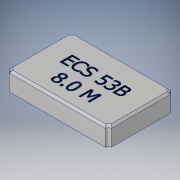
# Autodesk Inventor part: Crystal_ECX-42
Saved by Autodesk Inventor 2018 (Build 220112000, 112)
## iProperties
Created: 2016-08-15
Part Number: Crystal_ECX-42
Material: Aluminum 6061
Document SubType Name: Modeling
Designer: Bradley
Density: 2.7 g/cm^3
Appearance: Aluminum - Flat
Author: Bradley
Autodesk Inventor part; units mm, degrees
ref_plane "YZ Plane" through (0, 0, 0) normal (1, 0, 0) x (0, 1, 0)
ref_plane "XZ Plane" through (0, 0, 0) normal (0, 1, 0) x (-1, 0, 0)
ref_plane "XY Plane" through (0, 0, 0) normal (0, 0, 1) x (1, 0, 0)
sketch "Sketch1" plane through (0, 0, 0) normal (0, 1, 0) x (-1, 0, 0)
  line L0 (-2.5, 1.6) -> (2.5, 1.6)
  line L1 (2.5, 1.6) -> (2.5, -1.6)
  line L2 (2.5, -1.6) -> (-2.5, -1.6)
  line L3 (-2.5, -1.6) -> (-2.5, 1.6)
  line L4 (-2.5, 1.6) -> (2.5, -1.6) construction
  line L5 (2.5, 1.6) -> (-2.5, -1.6) construction
  arc A0 (2.5, -1.45) -> (2.35, -1.6) centre (2.5, -1.6) ccw
  arc A1 (-2.35, -1.6) -> (-2.5, -1.45) centre (-2.5, -1.6) ccw
  arc A2 (-2.5, 1.45) -> (-2.35, 1.6) centre (-2.5, 1.6) ccw
  arc A3 (2.35, 1.6) -> (2.5, 1.45) centre (2.5, 1.6) ccw
  point P0 (0, 0)
  dimension "d0" = 5
  dimension "d1" = 3.2
  dimension "d4" = 0.15
  constraints: 12 end point, 8 point on circle, 8 point on line, 4 centre point, 4 coincident, 3 equal radius, 2 midpoint, 2 parallel, 1 horizontal, 1 perpendicular
  measures "d0" distance of L1.end L2.end
  measures "d1" distance of L0.end L1.end
  measures "d4" radius of A0
extrude "Extrusion1" add sketch "Sketch1" along normal mid plane 0.9 contours L0 A3 L1 A0 L2 A1 L3 A2
chamfer "Chamfer1" distance 0.1 angle 45 8 edges at (0, 0.45, 1.6) (-2.3939, 0.45, 1.4939) (-2.5, 0.45, 0) (-2.3939, 0.45, -1.4939) (0, 0.45, -1.6) (2.3939, 0.45, -1.4939) (2.5, 0.45, 0) (2.3939, 0.45, 1.4939)
sketch "Sketch2" plane through (0, -0.45, 0) normal (0, -1, 0) x (1, 0, 0)
  line L0 (-2.5, 1.45) -> (-2.5, -1.45) projected
  arc A0 (-2.35, -1.6) -> (-2.5, -1.45) centre (-2.5, -1.6) ccw projected
  line L1 (-2.35, -1.6) -> (2.35, -1.6) projected
  arc A1 (2.5, -1.45) -> (2.35, -1.6) centre (2.5, -1.6) ccw projected
  line L2 (2.5, -1.45) -> (2.5, 1.45) projected
  arc A2 (2.35, 1.6) -> (2.5, 1.45) centre (2.5, 1.6) ccw projected
  line L3 (2.35, 1.6) -> (-2.35, 1.6) projected
  arc A3 (-2.5, 1.45) -> (-2.35, 1.6) centre (-2.5, 1.6) ccw projected
  arc A4 (-2.35, -1.6) -> (-2.5, -1.45) centre (-2.5, -1.6) ccw projected
  line L4 (-2.4612, -1.4551) -> (-2.4, -1.3939)
  line L5 (-2.4, 1.3939) -> (-2.4612, 1.4551)
  arc A5 (-2.5, 1.45) -> (-2.35, 1.6) centre (-2.5, 1.6) ccw projected
  line L6 (-2.3551, 1.5612) -> (-2.2939, 1.5)
  line L7 (-2.2939, 1.5) -> (-1.3, 1.5)
  line L8 (-1.3, -1.5) -> (-2.2939, -1.5)
  line L9 (-2.2939, -1.5) -> (-2.3551, -1.5612)
  arc A6 (2.35, 1.6) -> (2.5, 1.45) centre (2.5, 1.6) ccw projected
  line L10 (2.3551, 1.5612) -> (2.2939, 1.5)
  line L11 (2.2939, 1.5) -> (1.3, 1.5)
  line L12 (1.3, -1.5) -> (2.2939, -1.5)
  line L13 (2.2939, -1.5) -> (2.3551, -1.5612)
  arc A7 (2.5, -1.45) -> (2.35, -1.6) centre (2.5, -1.6) ccw projected
  line L14 (2.4612, -1.4551) -> (2.4, -1.3939)
  line L15 (2.4, 1.3939) -> (2.4612, 1.4551)
  line L16 (-2.5, 1.6) -> (-2.3939, 1.4939) construction
  line L17 (2.35, 1.6) -> (-2.35, 1.6) construction
  line L18 (-2.5, -1.6) -> (-2.3939, -1.4939) construction
  line L19 (-2.4, 1.3939) -> (-2.4, 0.7)
  line L20 (-2.4, 0.7) -> (-1.3, 0.7)
  line L21 (-1.3, 0.7) -> (-1.3, 1.5)
  line L22 (-2.4, -1.3939) -> (-2.4, -0.7)
  line L23 (-2.4, -0.7) -> (-1.3, -0.7)
  line L24 (-1.3, -0.7) -> (-1.3, -1.5)
  line L25 (2.4, -1.3939) -> (2.4, -0.7)
  line L26 (2.4, -0.7) -> (1.3, -0.7)
  line L27 (1.3, -0.7) -> (1.3, -1.5)
  line L28 (2.4, 1.3939) -> (2.4, 0.7)
  line L29 (2.4, 0.7) -> (1.3, 0.7)
  line L30 (1.3, 1.5) -> (1.3, 0.7)
  point P0 (0, 0)
  dimension "d9" = 0.15
  dimension "d17" = 0.8
  dimension "d20" = 1.1
  dimension "d22" = 0.1
  constraints: 52 end point, 15 equal length, 15 point on circle, 9 point on line, 8 parallel, 8 perpendicular, 1 collinear, 1 vertical, 1 other
  measures "d9" distance between parallel lines of L5 L6
  measures "d17" distance of L11.end L29.end
  measures "d20" distance of L28.end L29.end
  measures "d22" distance between parallel lines of L0 L19
sketch "Sketch3" plane through (0, 0.45, 0) normal (0, 1, 0) x (1, 0, 0)
  line L0 (-2.2709, 1.5) -> (2.2709, 1.5) projected
  arc A0 (-2.4, 1.3709) -> (-2.2709, 1.5) centre (-2.5, 1.6) ccw projected
  line L1 (-2.4, -1.3709) -> (-2.4, 1.3709) projected
  arc A1 (-2.2709, -1.5) -> (-2.4, -1.3709) centre (-2.5, -1.6) ccw projected
  line L2 (2.2709, -1.5) -> (-2.2709, -1.5) projected
  arc A2 (2.4, -1.3709) -> (2.2709, -1.5) centre (2.5, -1.6) ccw projected
  line L3 (2.4, 1.3709) -> (2.4, -1.3709) projected
  arc A3 (2.2709, 1.5) -> (2.4, 1.3709) centre (2.5, 1.6) ccw projected
  line L4 (2.4, 1.3709) -> (2.4, -1.3709) construction
  line L5 (2.4, 0) -> (-2.4, 0) construction
  line L6 (-1.4703, 0) -> (-1.4703, 0.6)
  line L7 (-1.4703, 0.6) -> (-1.095, 0.6)
  line L8 (-1.095, 0.6) -> (-1.095, 0.529)
  line L9 (-1.095, 0.529) -> (-1.3906, 0.529)
  line L10 (-1.3906, 0.529) -> (-1.3906, 0.3647)
  line L11 (-1.3906, 0.3647) -> (-1.1149, 0.3647)
  line L12 (-1.1149, 0.3647) -> (-1.1149, 0.2937)
  line L13 (-1.1149, 0.2937) -> (-1.3906, 0.2937)
  line L14 (-1.3906, 0.2937) -> (-1.3906, 0.071)
  line L15 (-1.3906, 0.071) -> (-1.095, 0.071)
  line L16 (-1.095, 0.071) -> (-1.095, 0)
  line L17 (-1.095, 0) -> (-1.4703, 0)
  spline S0 degree 2 poles (-0.7731, -0.0107) (-0.8314, -0.0107) (-0.9301, 0.0287) (-0.9661, 0.0681) knots 0 0 0 1 2 2 2
  spline S1 degree 2 poles (-0.9661, 0.0681) (-1.0021, 0.107) (-1.0415, 0.2237) (-1.0415, 0.2995) knots 0 0 0 1 2 2 2
  spline S2 degree 2 poles (-1.0415, 0.2995) (-1.0415, 0.3749) (-1.0031, 0.4867) (-0.9666, 0.528) knots 0 0 0 1 2 2 2
  spline S3 degree 2 poles (-0.9666, 0.528) (-0.9306, 0.5684) (-0.8324, 0.6107) (-0.7716, 0.6107) knots 0 0 0 1 2 2 2
  spline S4 degree 2 poles (-0.7716, 0.6107) (-0.7415, 0.6107) (-0.6885, 0.6019) (-0.6661, 0.5951) knots 0 0 0 1 2 2 2
  spline S5 degree 2 poles (-0.6661, 0.5951) (-0.6467, 0.5888) (-0.6063, 0.5708) (-0.5864, 0.5601) knots 0 0 0 1 2 2 2
  line L18 (-0.5864, 0.5601) -> (-0.5864, 0.4639)
  line L19 (-0.5864, 0.4639) -> (-0.5927, 0.4639)
  spline S6 degree 2 poles (-0.5927, 0.4639) (-0.6034, 0.4736) (-0.6365, 0.5008) (-0.6603, 0.5139) knots 0 0 0 1 2 2 2
  spline S7 degree 2 poles (-0.6603, 0.5139) (-0.6831, 0.5266) (-0.7371, 0.5426) (-0.7721, 0.5426) knots 0 0 0 1 2 2 2
  spline S8 degree 2 poles (-0.7721, 0.5426) (-0.8105, 0.5426) (-0.8791, 0.511) (-0.9049, 0.4809) knots 0 0 0 1 2 2 2
  spline S9 degree 2 poles (-0.9049, 0.4809) (-0.9301, 0.4502) (-0.9583, 0.3574) (-0.9583, 0.2995) knots 0 0 0 1 2 2 2
  spline S10 degree 2 poles (-0.9583, 0.2995) (-0.9583, 0.2378) (-0.9287, 0.1488) (-0.9029, 0.1182) knots 0 0 0 1 2 2 2
  spline S11 degree 2 poles (-0.9029, 0.1182) (-0.8776, 0.0885) (-0.81, 0.0583) (-0.7721, 0.0583) knots 0 0 0 1 2 2 2
  spline S12 degree 2 poles (-0.7721, 0.0583) (-0.7376, 0.0583) (-0.6788, 0.0754) (-0.6559, 0.088) knots 0 0 0 1 2 2 2
  spline S13 degree 2 poles (-0.6559, 0.088) (-0.634, 0.1006) (-0.6015, 0.1269) (-0.5922, 0.1361) knots 0 0 0 1 2 2 2
  line L20 (-0.5922, 0.1361) -> (-0.5864, 0.1361)
  line L21 (-0.5864, 0.1361) -> (-0.5864, 0.0408)
  spline S14 degree 2 poles (-0.5864, 0.0408) (-0.6063, 0.0316) (-0.6413, 0.0146) (-0.6661, 0.0068) knots 0 0 0 1 2 2 2
  spline S15 degree 2 poles (-0.6661, 0.0068) (-0.6924, -0.0019) (-0.7371, -0.0107) (-0.7731, -0.0107) knots 0 0 0 1 2 2 2
  spline S16 degree 2 poles (-0.3447, -0.0107) (-0.4099, -0.0107) (-0.5013, 0.0165) (-0.5417, 0.036) knots 0 0 0 1 2 2 2
  line L22 (-0.5417, 0.036) -> (-0.5417, 0.1361)
  line L23 (-0.5417, 0.1361) -> (-0.5358, 0.1361)
  spline S17 degree 2 poles (-0.5358, 0.1361) (-0.4964, 0.0992) (-0.3968, 0.0583) (-0.3506, 0.0583) knots 0 0 0 1 2 2 2
  spline S18 degree 2 poles (-0.3506, 0.0583) (-0.2844, 0.0583) (-0.2169, 0.1133) (-0.2169, 0.1585) knots 0 0 0 1 2 2 2
  spline S19 degree 2 poles (-0.2169, 0.1585) (-0.2169, 0.1945) (-0.2524, 0.2392) (-0.2908, 0.2504) knots 0 0 0 1 2 2 2
  spline S20 degree 2 poles (-0.2908, 0.2504) (-0.3185, 0.2582) (-0.3647, 0.2689) (-0.3992, 0.2776) knots 0 0 0 1 2 2 2
  spline S21 degree 2 poles (-0.3992, 0.2776) (-0.4303, 0.2859) (-0.4794, 0.3107) (-0.4984, 0.3306) knots 0 0 0 1 2 2 2
  spline S22 degree 2 poles (-0.4984, 0.3306) (-0.5169, 0.3506) (-0.5373, 0.4041) (-0.5373, 0.4391) knots 0 0 0 1 2 2 2
  spline S23 degree 2 poles (-0.5373, 0.4391) (-0.5373, 0.512) (-0.4235, 0.6107) (-0.3355, 0.6107) knots 0 0 0 1 2 2 2
  spline S24 degree 2 poles (-0.3355, 0.6107) (-0.2849, 0.6107) (-0.1955, 0.5908) (-0.1571, 0.5718) knots 0 0 0 1 2 2 2
  line L24 (-0.1571, 0.5718) -> (-0.1571, 0.4765)
  line L25 (-0.1571, 0.4765) -> (-0.1629, 0.4765)
  spline S25 degree 2 poles (-0.1629, 0.4765) (-0.1916, 0.5028) (-0.281, 0.5417) (-0.3301, 0.5417) knots 0 0 0 1 2 2 2
  spline S26 degree 2 poles (-0.3301, 0.5417) (-0.3856, 0.5417) (-0.4541, 0.4896) (-0.4541, 0.4473) knots 0 0 0 1 2 2 2
  spline S27 degree 2 poles (-0.4541, 0.4473) (-0.4541, 0.4094) (-0.4138, 0.3642) (-0.3759, 0.354) knots 0 0 0 1 2 2 2
  spline S28 degree 2 poles (-0.3759, 0.354) (-0.3506, 0.3472) (-0.2771, 0.3297) (-0.2528, 0.3224) knots 0 0 0 1 2 2 2
  spline S29 degree 2 poles (-0.2528, 0.3224) (-0.1911, 0.3034) (-0.1337, 0.2271) (-0.1337, 0.1712) knots 0 0 0 1 2 2 2
  spline S30 degree 2 poles (-0.1337, 0.1712) (-0.1337, 0.1357) (-0.1624, 0.0676) (-0.1882, 0.0438) knots 0 0 0 1 2 2 2
  spline S31 degree 2 poles (-0.1882, 0.0438) (-0.2169, 0.0175) (-0.2898, -0.0107) (-0.3447, -0.0107) knots 0 0 0 1 2 2 2
  spline S32 degree 2 poles (0.5519, 0.1906) (0.5519, 0.1473) (0.5241, 0.0734) (0.4989, 0.0462) knots 0 0 0 1 2 2 2
  spline S33 degree 2 poles (0.4989, 0.0462) (0.4736, 0.019) (0.3982, -0.0126) (0.3515, -0.0126) knots 0 0 0 1 2 2 2
  spline S34 degree 2 poles (0.3515, -0.0126) (0.3088, -0.0126) (0.2251, 0.0063) (0.1945, 0.0214) knots 0 0 0 1 2 2 2
  line L26 (0.1945, 0.0214) -> (0.1945, 0.1065)
  line L27 (0.1945, 0.1065) -> (0.2003, 0.1065)
  spline S35 degree 2 poles (0.2003, 0.1065) (0.2096, 0.0997) (0.2441, 0.0822) (0.265, 0.0744) knots 0 0 0 1 2 2 2
  spline S36 degree 2 poles (0.265, 0.0744) (0.2888, 0.0661) (0.3282, 0.0569) (0.353, 0.0569) knots 0 0 0 1 2 2 2
  spline S37 degree 2 poles (0.353, 0.0569) (0.3773, 0.0569) (0.423, 0.0744) (0.4395, 0.0934) knots 0 0 0 1 2 2 2
  spline S38 degree 2 poles (0.4395, 0.0934) (0.4546, 0.1113) (0.4702, 0.159) (0.4702, 0.1911) knots 0 0 0 1 2 2 2
  spline S39 degree 2 poles (0.4702, 0.1911) (0.4702, 0.2232) (0.4527, 0.264) (0.4361, 0.2776) knots 0 0 0 1 2 2 2
  spline S40 degree 2 poles (0.4361, 0.2776) (0.4191, 0.2927) (0.3686, 0.3053) (0.3379, 0.3053) knots 0 0 0 1 2 2 2
  spline S41 degree 2 poles (0.3379, 0.3053) (0.3049, 0.3053) (0.2392, 0.2951) (0.2193, 0.2908) knots 0 0 0 1 2 2 2
  line L28 (0.2193, 0.2908) -> (0.2193, 0.6)
  line L29 (0.2193, 0.6) -> (0.5485, 0.6)
  line L30 (0.5485, 0.6) -> (0.5485, 0.5295)
  line L31 (0.5485, 0.5295) -> (0.2966, 0.5295)
  line L32 (0.2966, 0.5295) -> (0.2966, 0.3695)
  spline S42 degree 2 poles (0.2966, 0.3695) (0.3112, 0.3715) (0.3394, 0.3729) (0.3511, 0.3729) knots 0 0 0 1 2 2 2
  spline S43 degree 2 poles (0.3511, 0.3729) (0.3972, 0.3729) (0.4609, 0.3579) (0.4901, 0.3355) knots 0 0 0 1 2 2 2
  spline S44 degree 2 poles (0.4901, 0.3355) (0.5198, 0.3131) (0.5519, 0.2451) (0.5519, 0.1906) knots 0 0 0 1 2 2 2
  spline S45 degree 2 poles (0.8003, 0.5431) (0.7784, 0.5431) (0.7352, 0.5324) (0.7143, 0.5241) knots 0 0 0 1 2 2 2
  spline S46 degree 2 poles (0.7143, 0.5241) (0.6948, 0.5159) (0.6661, 0.4984) (0.6549, 0.4906) knots 0 0 0 1 2 2 2
  line L33 (0.6549, 0.4906) -> (0.6501, 0.4906)
  line L34 (0.6501, 0.4906) -> (0.6501, 0.5757)
  spline S47 degree 2 poles (0.6501, 0.5757) (0.6763, 0.5898) (0.7663, 0.6126) (0.8066, 0.6126) knots 0 0 0 1 2 2 2
  spline S48 degree 2 poles (0.8066, 0.6126) (0.8475, 0.6126) (0.9083, 0.5961) (0.9331, 0.5786) knots 0 0 0 1 2 2 2
  spline S49 degree 2 poles (0.9331, 0.5786) (0.9593, 0.5596) (0.9865, 0.5047) (0.9865, 0.4677) knots 0 0 0 1 2 2 2
  spline S50 degree 2 poles (0.9865, 0.4677) (0.9865, 0.4182) (0.9214, 0.3433) (0.8757, 0.3335) knots 0 0 0 1 2 2 2
  line L35 (0.8757, 0.3335) -> (0.8757, 0.3277)
  spline S51 degree 2 poles (0.8757, 0.3277) (0.8947, 0.3238) (0.9379, 0.3063) (0.9564, 0.2888) knots 0 0 0 1 2 2 2
  spline S52 degree 2 poles (0.9564, 0.2888) (0.9749, 0.2718) (0.9982, 0.2173) (0.9982, 0.178) knots 0 0 0 1 2 2 2
  spline S53 degree 2 poles (0.9982, 0.178) (0.9982, 0.1376) (0.9705, 0.069) (0.9452, 0.0428) knots 0 0 0 1 2 2 2
  spline S54 degree 2 poles (0.9452, 0.0428) (0.919, 0.0156) (0.8446, -0.0126) (0.7974, -0.0126) knots 0 0 0 1 2 2 2
  spline S55 degree 2 poles (0.7974, -0.0126) (0.7522, -0.0126) (0.6637, 0.0092) (0.6335, 0.0243) knots 0 0 0 1 2 2 2
  line L36 (0.6335, 0.0243) -> (0.6335, 0.1094)
  line L37 (0.6335, 0.1094) -> (0.6394, 0.1094)
  spline S56 degree 2 poles (0.6394, 0.1094) (0.6647, 0.0909) (0.7502, 0.0569) (0.7925, 0.0569) knots 0 0 0 1 2 2 2
  spline S57 degree 2 poles (0.7925, 0.0569) (0.8173, 0.0569) (0.8669, 0.0724) (0.8835, 0.0904) knots 0 0 0 1 2 2 2
  spline S58 degree 2 poles (0.8835, 0.0904) (0.8995, 0.1084) (0.9165, 0.1512) (0.9165, 0.1838) knots 0 0 0 1 2 2 2
  spline S59 degree 2 poles (0.9165, 0.1838) (0.9165, 0.2164) (0.8976, 0.2587) (0.8806, 0.2708) knots 0 0 0 1 2 2 2
  spline S60 degree 2 poles (0.8806, 0.2708) (0.8635, 0.283) (0.8173, 0.2922) (0.7901, 0.2922) knots 0 0 0 1 2 2 2
  line L38 (0.7901, 0.2922) -> (0.7561, 0.2922)
  line L39 (0.7561, 0.2922) -> (0.7561, 0.3588)
  line L40 (0.7561, 0.3588) -> (0.7828, 0.3588)
  spline S61 degree 2 poles (0.7828, 0.3588) (0.8368, 0.3588) (0.9049, 0.4104) (0.9049, 0.4595) knots 0 0 0 1 2 2 2
  spline S62 degree 2 poles (0.9049, 0.4595) (0.9049, 0.4823) (0.8874, 0.5149) (0.8733, 0.5246) knots 0 0 0 1 2 2 2
  spline S63 degree 2 poles (0.8733, 0.5246) (0.8582, 0.5348) (0.8212, 0.5431) (0.8003, 0.5431) knots 0 0 0 1 2 2 2
  spline S64 degree 2 poles (1.5126, 0.1843) (1.5126, 0.1395) (1.4786, 0.071) (1.4504, 0.0486) knots 0 0 0 1 2 2 2
  spline S65 degree 2 poles (1.4504, 0.0486) (1.4164, 0.0224) (1.3391, 0) (1.2778, 0) knots 0 0 0 1 2 2 2
  line L41 (1.2778, 0) -> (1.1057, 0)
  line L42 (1.1057, 0) -> (1.1057, 0.6)
  line L43 (1.1057, 0.6) -> (1.2647, 0.6)
  spline S66 degree 2 poles (1.2647, 0.6) (1.3288, 0.6) (1.393, 0.5917) (1.4222, 0.5757) knots 0 0 0 1 2 2 2
  spline S67 degree 2 poles (1.4222, 0.5757) (1.4548, 0.5587) (1.4844, 0.5028) (1.4844, 0.4648) knots 0 0 0 1 2 2 2
  spline S68 degree 2 poles (1.4844, 0.4648) (1.4844, 0.4225) (1.4397, 0.3554) (1.4003, 0.3365) knots 0 0 0 1 2 2 2
  line L44 (1.4003, 0.3365) -> (1.4003, 0.3335)
  spline S69 degree 2 poles (1.4003, 0.3335) (1.4538, 0.319) (1.5126, 0.2417) (1.5126, 0.1843) knots 0 0 0 1 2 2 2
  spline S70 degree 2 poles (1.4295, 0.1809) (1.4295, 0.2149) (1.41, 0.2587) (1.3809, 0.2742) knots 0 0 0 1 2 2 2
  spline S71 degree 2 poles (1.3809, 0.2742) (1.3619, 0.284) (1.3172, 0.2898) (1.2759, 0.2898) knots 0 0 0 1 2 2 2
  line L45 (1.2759, 0.2898) -> (1.1854, 0.2898)
  line L46 (1.1854, 0.2898) -> (1.1854, 0.0681)
  line L47 (1.1854, 0.0681) -> (1.2501, 0.0681)
  spline S72 degree 2 poles (1.2501, 0.0681) (1.3026, 0.0681) (1.3629, 0.0778) (1.3862, 0.0934) knots 0 0 0 1 2 2 2
  spline S73 degree 2 poles (1.3862, 0.0934) (1.4086, 0.1094) (1.4295, 0.1493) (1.4295, 0.1809) knots 0 0 0 1 2 2 2
  spline S74 degree 2 poles (1.4013, 0.4536) (1.4013, 0.475) (1.3867, 0.5071) (1.3707, 0.5164) knots 0 0 0 1 2 2 2
  spline S75 degree 2 poles (1.3707, 0.5164) (1.3512, 0.5271) (1.3041, 0.5319) (1.2618, 0.5319) knots 0 0 0 1 2 2 2
  line L48 (1.2618, 0.5319) -> (1.1854, 0.5319)
  line L49 (1.1854, 0.5319) -> (1.1854, 0.3564)
  line L50 (1.1854, 0.3564) -> (1.2759, 0.3564)
  spline S76 degree 2 poles (1.2759, 0.3564) (1.3133, 0.3564) (1.3488, 0.3642) (1.3677, 0.3763) knots 0 0 0 1 2 2 2
  spline S77 degree 2 poles (1.3677, 0.3763) (1.3862, 0.388) (1.4013, 0.4254) (1.4013, 0.4536) knots 0 0 0 1 2 2 2
  spline S78 degree 2 poles (-0.7969, -1.0054) (-0.8417, -1.0054) (-0.9151, -0.9787) (-0.9408, -0.9539) knots 0 0 0 1 2 2 2
  spline S79 degree 2 poles (-0.9408, -0.9539) (-0.9661, -0.9296) (-0.9924, -0.8634) (-0.9924, -0.826) knots 0 0 0 1 2 2 2
  spline S80 degree 2 poles (-0.9924, -0.826) (-0.9924, -0.7774) (-0.9404, -0.6957) (-0.8908, -0.6714) knots 0 0 0 1 2 2 2
  line L51 (-0.8908, -0.6714) -> (-0.8908, -0.6689)
  spline S81 degree 2 poles (-0.8908, -0.6689) (-0.935, -0.6432) (-0.9778, -0.5819) (-0.9778, -0.5362) knots 0 0 0 1 2 2 2
  spline S82 degree 2 poles (-0.9778, -0.5362) (-0.9778, -0.4686) (-0.8757, -0.3782) (-0.7969, -0.3782) knots 0 0 0 1 2 2 2
  spline S83 degree 2 poles (-0.7969, -0.3782) (-0.7152, -0.3782) (-0.6165, -0.4637) (-0.6165, -0.5308) knots 0 0 0 1 2 2 2
  spline S84 degree 2 poles (-0.6165, -0.5308) (-0.6165, -0.5712) (-0.6637, -0.65) (-0.7079, -0.6723) knots 0 0 0 1 2 2 2
  line L52 (-0.7079, -0.6723) -> (-0.7079, -0.6748)
  spline S85 degree 2 poles (-0.7079, -0.6748) (-0.6554, -0.6991) (-0.6015, -0.7691) (-0.6015, -0.8245) knots 0 0 0 1 2 2 2
  spline S86 degree 2 poles (-0.6015, -0.8245) (-0.6015, -0.9014) (-0.7133, -1.0054) (-0.7969, -1.0054) knots 0 0 0 1 2 2 2
  spline S87 degree 2 poles (-0.6841, -0.8323) (-0.6841, -0.7954) (-0.7133, -0.7516) (-0.7546, -0.7292) knots 0 0 0 1 2 2 2
  spline S88 degree 2 poles (-0.7546, -0.7292) (-0.7682, -0.7214) (-0.8139, -0.7035) (-0.8426, -0.6918) knots 0 0 0 1 2 2 2
  spline S89 degree 2 poles (-0.8426, -0.6918) (-0.8757, -0.7137) (-0.9112, -0.7788) (-0.9112, -0.8202) knots 0 0 0 1 2 2 2
  spline S90 degree 2 poles (-0.9112, -0.8202) (-0.9112, -0.8746) (-0.8455, -0.9456) (-0.7959, -0.9456) knots 0 0 0 1 2 2 2
  spline S91 degree 2 poles (-0.7959, -0.9456) (-0.7454, -0.9456) (-0.6841, -0.8848) (-0.6841, -0.8323) knots 0 0 0 1 2 2 2
  spline S92 degree 2 poles (-0.6953, -0.5318) (-0.6953, -0.4915) (-0.7493, -0.4375) (-0.7974, -0.4375) knots 0 0 0 1 2 2 2
  spline S93 degree 2 poles (-0.7974, -0.4375) (-0.8412, -0.4375) (-0.8971, -0.4856) (-0.8971, -0.527) knots 0 0 0 1 2 2 2
  spline S94 degree 2 poles (-0.8971, -0.527) (-0.8971, -0.5566) (-0.8684, -0.5979) (-0.8397, -0.6145) knots 0 0 0 1 2 2 2
  spline S95 degree 2 poles (-0.8397, -0.6145) (-0.8276, -0.6213) (-0.776, -0.6451) (-0.7551, -0.6519) knots 0 0 0 1 2 2 2
  spline S96 degree 2 poles (-0.7551, -0.6519) (-0.7201, -0.6252) (-0.6953, -0.5683) (-0.6953, -0.5318) knots 0 0 0 1 2 2 2
  line L53 (-0.3992, -0.9918) -> (-0.4955, -0.9918)
  line L54 (-0.4955, -0.9918) -> (-0.4955, -0.877)
  line L55 (-0.4955, -0.877) -> (-0.3992, -0.877)
  line L56 (-0.3992, -0.877) -> (-0.3992, -0.9918)
  spline S97 degree 2 poles (0.0953, -0.6918) (0.0953, -0.8532) (0.0015, -1.0044) (-0.0963, -1.0044) knots 0 0 0 1 2 2 2
  spline S98 degree 2 poles (-0.0963, -1.0044) (-0.1955, -1.0044) (-0.2883, -0.8503) (-0.2883, -0.6923) knots 0 0 0 1 2 2 2
  spline S99 degree 2 poles (-0.2883, -0.6923) (-0.2883, -0.5299) (-0.1945, -0.3796) (-0.0963, -0.3796) knots 0 0 0 1 2 2 2
  spline S100 degree 2 poles (-0.0963, -0.3796) (0.0024, -0.3796) (0.0953, -0.5352) (0.0953, -0.6918) knots 0 0 0 1 2 2 2
  spline S101 degree 2 poles (-0.0078, -0.8746) (0.0039, -0.8449) (0.0136, -0.7535) (0.0136, -0.6918) knots 0 0 0 1 2 2 2
  spline S102 degree 2 poles (0.0136, -0.6918) (0.0136, -0.63) (0.0039, -0.5391) (-0.0083, -0.5085) knots 0 0 0 1 2 2 2
  spline S103 degree 2 poles (-0.0083, -0.5085) (-0.0204, -0.4778) (-0.0627, -0.4462) (-0.0963, -0.4462) knots 0 0 0 1 2 2 2
  spline S104 degree 2 poles (-0.0963, -0.4462) (-0.1298, -0.4462) (-0.1731, -0.4778) (-0.1857, -0.5095) knots 0 0 0 1 2 2 2
  spline S105 degree 2 poles (-0.1857, -0.5095) (-0.1979, -0.5401) (-0.2066, -0.6334) (-0.2066, -0.6923) knots 0 0 0 1 2 2 2
  spline S106 degree 2 poles (-0.2066, -0.6923) (-0.2066, -0.7555) (-0.1989, -0.8401) (-0.1862, -0.8731) knots 0 0 0 1 2 2 2
  spline S107 degree 2 poles (-0.1862, -0.8731) (-0.1746, -0.9043) (-0.1313, -0.9378) (-0.0963, -0.9378) knots 0 0 0 1 2 2 2
  spline S108 degree 2 poles (-0.0963, -0.9378) (-0.0632, -0.9378) (-0.0199, -0.9062) (-0.0078, -0.8746) knots 0 0 0 1 2 2 2
  line L57 (0.9613, -0.9918) -> (0.8815, -0.9918)
  line L58 (0.8815, -0.9918) -> (0.8815, -0.4749)
  line L59 (0.8815, -0.4749) -> (0.725, -0.8265)
  line L60 (0.725, -0.8265) -> (0.6763, -0.8265)
  line L61 (0.6763, -0.8265) -> (0.5212, -0.4749)
  line L62 (0.5212, -0.4749) -> (0.5212, -0.9918)
  line L63 (0.5212, -0.9918) -> (0.4468, -0.9918)
  line L64 (0.4468, -0.9918) -> (0.4468, -0.3918)
  line L65 (0.4468, -0.3918) -> (0.5558, -0.3918)
  line L66 (0.5558, -0.3918) -> (0.7055, -0.7258)
  line L67 (0.7055, -0.7258) -> (0.8504, -0.3918)
  line L68 (0.8504, -0.3918) -> (0.9613, -0.3918)
  line L69 (0.9613, -0.3918) -> (0.9613, -0.9918)
  point P0 (0, 0)
  constraints: 3 midpoint, 2 end point, 1 horizontal, 1 perpendicular
extrude "Extrusion3" add sketch "Sketch3" along normal blind 0.01 contours L6 L7 L8 L9 L10 L11 L12 L13 L14 L15 L16 L17 | S0 S1 S2 S3 S4 S5 L18 L19 S6 S7 S8 S9 S10 S11 S12 S13 L20 L21 S14 S15 | S16 L22 L23 S17 S18 S19 S20 S21 S22 S23 S24 L24 L25 S25 S26 S27 S28 S29 S30 S31 | S32 S33 S34 L26 L27 S35 S36 S37 S38 S39 S40 S41 L28 L29 L30 L31 L32 S42 S43 S44 | S45 S46 L33 L34 S47 S48 S49 S50 L35 S51 S52 S53 S54 S55 L36 L37 S56 S57 S58 S59 S60 L38 L39 L40 S61 S62 S63 | S64 S65 L41 L42 L43 S66 S67 S68 L44 S69 | S78 S79 S80 L51 S81 S82 S83 S84 L52 S85 S86 | L53 L54 L55 L56 | S97 S98 S99 S100 | L57 L58 L59 L60 L61 L62 L63 L64 L65 L66 L67 L68 L69
extrude "Extrusion4" add sketch "Sketch2" along normal blind 0.01 contours A3 L6 L7 L21 L20 L19 L5 | L4 L22 L23 L24 L8 L9 A0 | A2 L15 L28 L29 L30 L11 L10 | L13 L12 L27 L26 L25 L14 A1
body "Solid1"
